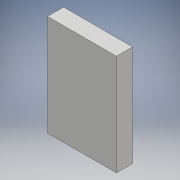
# Autodesk Inventor part: Tronco
Saved by Autodesk Inventor 2018 (Build 220112000, 112)
## iProperties
Created: 2020-03-08
Part Number: Tronco
Material: Generic
Document SubType Name: Modeling
Designer: GonzaloDiaz
Density: 1 g/cm^3
Appearance: Default
Author: GonzaloDiaz
Autodesk Inventor part; units mm, degrees
ref_plane "YZ Plane" through (0, 0, 0) normal (1, 0, 0) x (0, 1, 0)
ref_plane "XZ Plane" through (0, 0, 0) normal (0, 1, 0) x (-1, 0, 0)
ref_plane "XY Plane" through (0, 0, 0) normal (0, 0, 1) x (1, 0, 0)
sketch "Sketch1" plane through (0, 0, 0) normal (0, 1, 0) x (-1, 0, 0)
  line L0 (0, 0) -> (150, 0)
  line L1 (150, 0) -> (150, -220)
  line L2 (150, -220) -> (0, -220)
  line L3 (0, -220) -> (0, 0)
  dimension "d0" = 150
  dimension "d1" = 220
  constraints: 8 end point, 2 parallel, 1 horizontal, 1 perpendicular
  measures "d0" distance of L1.end L2.end
  measures "d1" distance of L0.end L1.end
extrude "Extrusion1" add sketch "Sketch1" along normal blind 5
sketch "Sketch3" plane through (0, 5, 0) normal (0, 1, 0) x (1, 0, 0)
  line L0 (-150, 0) -> (0, 0) projected
  line L1 (0, 0) -> (0, 220) projected
  line L2 (-150, 0) -> (0, 0)
  line L3 (0, 0) -> (0, 220)
  line L4 (0, 220) -> (-150, 220)
  line L5 (-150, 220) -> (-150, 0)
  line L6 (-145, 5) -> (-5, 5)
  line L7 (-5, 5) -> (-5, 215)
  line L8 (-5, 215) -> (-145, 215)
  line L9 (-145, 215) -> (-145, 5)
  dimension "d4" = 5
  dimension "d5" = 5
  dimension "d6" = 5
  dimension "d7" = 5
  constraints: 16 end point, 4 parallel, 2 horizontal, 2 perpendicular
  measures "d4" distance between parallel lines of L4 L8
  measures "d5" distance between parallel lines of L0 L6
  measures "d6" distance between parallel lines of L5 L9
  measures "d7" distance between parallel lines of L1 L7
extrude "Extrusion2" add sketch "Sketch3" along normal blind 30
body "Solid1"
